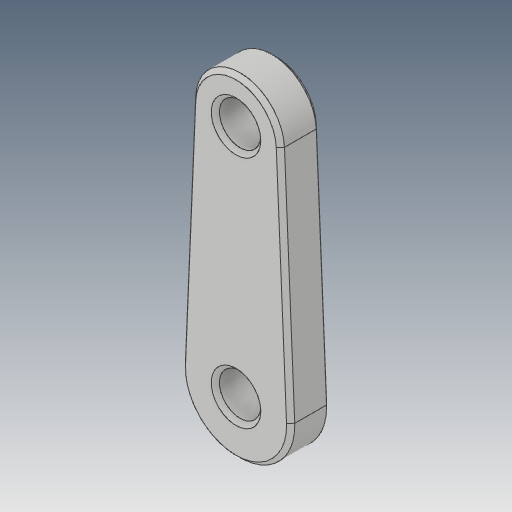
# Autodesk Inventor part: hinge_guid_a
Saved by Autodesk Inventor 2018 (Build 220112000, 112)
## iProperties
Created: 2019-01-31
Part Number: hinge_guid_a
Material: Generic
Document SubType Name: Modeling
Designer: Tsche
Density: 1 g/cm^3
Appearance: Default
Author: Tsche
Autodesk Inventor part; units mm, degrees
ref_plane "YZ Plane" through (0, 0, 0) normal (1, 0, 0) x (0, 1, 0)
ref_plane "XZ Plane" through (0, 0, 0) normal (0, 1, 0) x (-1, 0, 0)
ref_plane "XY Plane" through (0, 0, 0) normal (0, 0, 1) x (1, 0, 0)
sketch "Sketch1" plane through (0, 0, 0) normal (0, 0, 1) x (1, 0, 0)
  circle A0 centre (0, 0) radius 1.5125
  circle A1 centre (0, 17.145) radius 1.5125
  line L0 (0, 0) -> (0, 17.145) construction
  arc A2 (-3.9962, 0.175) -> (3.9962, 0.175) centre (0, 0) ccw
  arc A3 (3.2469, 17.2872) -> (-3.2469, 17.2872) centre (0, 17.145) ccw
  line L1 (-3.2469, 17.2872) -> (-3.9962, 0.175)
  line L2 (3.9962, 0.175) -> (3.2469, 17.2872)
  dimension "d2" = 17.145
  dimension "d3" = 4
  dimension "d4" = 3.025
  dimension "d12" = 3.25
  constraints: 6 end point, 5 point on circle, 4 centre point, 4 tangent, 2 concentric, 1 coincident, 1 equal radius, 1 vertical
  measures "d2" distance of L0.start L0.end
  measures "d3" radius of A2
  measures "d4" diameter of A0
  measures "d12" radius of A3
extrude "Extrusion1" add sketch "Sketch1" along normal mid plane 2.925
sketch "Sketch2" plane through (0, 0, 1.4625) normal (0, 0, 1) x (1, 0, 0)
  circle A0 centre (0, 0) radius 1.5125 projected
  arc A1 (-3.9962, 0.175) -> (3.9962, 0.175) centre (0, 0) ccw construction
  circle A2 centre (0, 0) radius 4
  constraints: 1 centre point, 1 coincident, 1 concentric
extrude "Extrusion2" [suppressed]
chamfer "Chamfer1" distance 0.3 angle 45 12 edges at (3.6215, 8.7311, -1.4625) (0, -4, -1.4625) (-3.6215, 8.7311, -1.4625) (0, 20.395, -1.4625) (-1.5125, 17.145, -1.4625) (-1.5125, 17.145, 1.4625) (3.6215, 8.7311, 1.4625) (0, 20.395, 1.4625) (-3.6215, 8.7311, 1.4625) (0, -4, 1.4625) (-1.5125, 0, -1.4625) (-1.5125, 0, 1.4625)
equation "\"d2\" = hinge_guid_length_a"
equation "\"d3\" = 0.5 * finger_thickness"
equation "\"d4\" = bore_clearance"
equation "\"d12\" = 0.5 * bar_diameter"
equation "\"d5\" = hinge_thickness - finger_link_clearence"
equation "\"d9\" = champfer"
equation "\"bore_press\" = 2.925"
equation "\"bore_clearance\" = 3.025"
equation "\"hinge_act_length_ab\" = 11.049"
equation "\"hinge_act_length_bc\" = 16.66875"
equation "\"bar_diameter\" = 6.5"
equation "\"hinge_thickness\" = 3"
equation "\"finger_width\" = 25"
equation "\"finger_thickness\" = 8"
equation "\"finger_part_A_length\" = 42.8625"
equation "\"finger_part_B_length\" = 28.575"
equation "\"finger_link_width\" = 3.5"
equation "\"finger_link_clearence\" = 0.075"
equation "\"tol\" = 0.5 * finger_link_clearence"
equation "\"link_tol\" = 0.254"
equation "\"bar_thickness\" = 4"
equation "\"bar_width\" = 7"
equation "\"hinge_dist_sym_plane\" = 4"
equation "\"hinge_act_length_c\" = 7.62"
equation "\"hinge_act_length_a\" = 21.43125"
equation "\"hinge_guid_length_c\" = 9.525"
equation "\"hinge_guid_length_bc\" = 9.525"
equation "\"hinge_guid_length_ab\" = 17.145"
equation "\"hinge_guid_length_a\" = 17.145"
equation "\"bar_length_bc\" = finger_part_B_length"
equation "\"bar_act_length_ab\" = 40.48125"
equation "\"bar_guid_length_ab\" = 43.275"
equation "\"champfer\" = 0.3"
equation "\"fillet\" = 0.4"
equation "\"dist_finger_BC\" = 56.5"
equation "\"gear_diameter\" = 14"
equation "\"hinge_point\" = 15"
body "Solid1"
